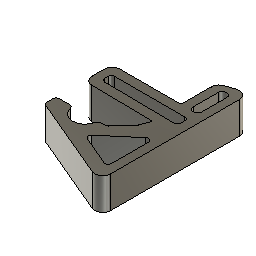
支架 v9 (Autodesk Fusion 360 design; units mm, degrees)
Autodesk Fusion 360 part; units mm, degrees
sketch "草图1" plane through (0, 0, 0) normal (0, 0, 1) x (1, 0, 0) in component "support"
  line L0 (40.3306, 33.6594) -> (40.3306, -61.561)
  line L1 (40.3306, -61.561) -> (-18.6734, -36.5899)
  line L2 (-18.6734, -36.5899) -> (-18.6734, 5.8967)
  line L3 (-18.6734, 5.8967) -> (24.5506, 5.8967)
  line L4 (24.5506, 5.8967) -> (24.5506, 28.4577)
  line L5 (24.5506, 28.4577) -> (40.3306, 33.6594)
  line L6 (35.2823, 8.3501) -> (35.2823, 23.9544)
  arc A0 (35.2823, 23.9544) -> (29.8253, 23.9544) centre (32.5538, 23.9544) ccw
  line L7 (29.8253, 23.9544) -> (29.8253, 8.3501)
  arc A1 (29.8253, 8.3501) -> (35.2823, 8.3501) centre (32.5538, 8.3501) ccw
  line L8 (32.5538, 5.6216) -> (32.5538, 26.6829) construction
  line L9 (-13.4908, -5.8932) -> (34.7153, -6.5796)
  line L10 (34.7153, -6.5796) -> (34.7153, 0.2419)
  line L11 (-18.6734, -11.6226) -> (24.884, -12.2428)
  line L12 (24.884, -12.2428) -> (22.3355, -19.0792)
  line L13 (-7.9409, -29.2052) -> (-18.6734, -29.2052)
  line L14 (35, -20.4957) -> (35, -51.1893)
  line L15 (-13.4908, 0.2419) -> (-13.4908, -5.8932)
  line L16 (34.7153, 0.2419) -> (-13.4908, 0.2419)
  line L17 (35, -51.1893) -> (10.8843, -40.9833)
  line L18 (10.8843, -40.9833) -> (35, -20.4957)
  line L19 (12.9862, -29.3446) -> (22.3355, -19.0792)
  line L20 (12.9862, -29.3446) -> (7.5042, -29.3446)
  arc A2 (-7.9409, -29.2052) -> (7.5042, -29.3446) centre (-0.2208, -29.5486) ccw
  constraint parallel L2 L4
  constraint tangent L6 A0
  constraint tangent A0 L7
  constraint parallel L6 L7
  constraint tangent L7 A1
  constraint tangent L6 A1
  constraint midpoint A1 L8.start
  constraint midpoint A0 L8.end
  constraint vertical L10
  constraint coincident L2 L11.start
  constraint parallel L9 L11
  constraint coincident L2 L13.end
  constraint horizontal L13
  constraint perpendicular L13 L14
  constraint perpendicular L15 L16
  constraint parallel L1 L17
  constraint horizontal L20
  constraint parallel L3 L16
  constraint parallel L2 L15
  constraint vertical L0
  constraint vertical L6
  constraint vertical L4
extrude "拉伸4" add sketch "草图1" along normal blind 20 contours L0 L1 L2 L3 L4 L5 L11 L12 L13 L19 L20 A2 in component "support"
fillet "圆角22" radius 2 1 edges at (10.8843, -40.9833, 10) in component "support"
fillet "圆角23" radius 2 1 edges at (35, -51.1893, 10) in component "support"
fillet "圆角24" radius 2 1 edges at (35, -20.4957, 10) in component "support"
fillet "圆角25" radius 5 1 edges at (40.3306, -61.561, 10) in component "support"
fillet "圆角26" radius 5 1 edges at (40.3306, 33.6594, 10) in component "support"
fillet "圆角27" radius 5 1 edges at (24.5506, 28.4577, 10) in component "support"
fillet "圆角28" radius 2 1 edges at (24.5506, 5.8967, 10) in component "support"
fillet "圆角29" radius 5 2 edges at (-18.6734, 5.8967, 10) (-18.6734, -11.6226, 10) in component "support"
fillet "圆角30" radius 2 1 edges at (-18.6734, -29.2052, 10) in component "support"
fillet "圆角31" radius 2 1 edges at (-18.6734, -36.5899, 10) in component "support"
fillet "圆角32" radius 2 1 edges at (34.7153, 0.2419, 10) in component "support"
fillet "圆角33" radius 2 1 edges at (34.7153, -6.5796, 10) in component "support"
fillet "圆角34" radius 2 1 edges at (-13.4908, -5.8932, 10) in component "support"
fillet "圆角35" radius 2 1 edges at (-13.4908, 0.2419, 10) in component "support"
fillet "圆角36" radius 0.5 1 edges at (24.884, -12.2428, 10) in component "support"
fillet "圆角37" radius 1 1 edges at (22.3355, -19.0792, 10) in component "support"
fillet "圆角38" radius 2 1 edges at (12.9862, -29.3446, 10) in component "support"
fillet "圆角39" radius 3 1 edges at (-7.9409, -29.2052, 10) in component "support"
fillet "圆角40" radius 3 1 edges at (7.5042, -29.3446, 10) in component "support"
component "support" placed x (1, 0, 0) y (0, 1, 0) z (0, 0, 1) at (0, 0, 0)
